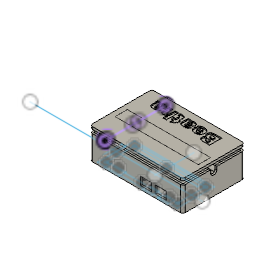
beatha (Autodesk Fusion 360 design; units mm, degrees)
Autodesk Fusion 360 part; units mm, degrees
note: some values were not read from the file. Chosen so that the rebuilt part matches the saved one: which face or edge a step refers to; which pieces of a blend or face edit are solid. Set by a fixed rule: which sketch regions a step uses.
sketch "pi w reference" plane through (0, 0, 0) normal (0, 1, 0) x (1, 0, 0)
  line L0 (-7.686, 3.5496) -> (57.314, 3.5496)
  line L1 (57.314, 3.5496) -> (57.314, -26.4504)
  line L2 (57.314, -26.4504) -> (-7.686, -26.4504)
  line L3 (-7.686, -26.4504) -> (-7.686, 3.5496)
  line L4 (-4.186, 0.0496) -> (53.814, 0.0496)
  line L5 (53.814, 0.0496) -> (53.814, -22.9504)
  line L6 (53.814, -22.9504) -> (-4.186, -22.9504)
  line L7 (-4.186, -22.9504) -> (-4.186, 0.0496)
  line L8 (24.814, 19.4382) -> (24.814, -12.339)
  line L9 (-77.996, -11.4504) -> (62.624, -11.4504)
  circle A0 centre (-4.186, 0.0496) radius 1.25
  circle A1 centre (-4.186, -22.9504) radius 1.25
  circle A2 centre (53.814, -22.9504) radius 1.25
  circle A3 centre (53.814, 0.0496) radius 1.25
  line L10 (-7.686, -3.9504) -> (-10.686, -3.9504)
  line L11 (-10.686, -3.9504) -> (-10.686, -18.9504)
  line L12 (-10.686, -18.9504) -> (-7.686, -18.9504) construction
  line L13 (-7.686, -18.9504) -> (-7.686, -3.9504)
  line L14 (-1.286, -21.9504) -> (10.714, -21.9504)
  line L15 (10.714, -21.9504) -> (10.714, -27.4504)
  line L16 (10.714, -27.4504) -> (-1.286, -27.4504)
  line L17 (-1.286, -27.4504) -> (-1.286, -21.9504)
  line L18 (29.714, -21.9504) -> (37.714, -21.9504)
  line L19 (37.714, -21.9504) -> (37.714, -27.4504)
  line L20 (37.714, -27.4504) -> (29.714, -27.4504)
  line L21 (29.714, -27.4504) -> (29.714, -21.9504)
  line L22 (42.314, -21.9504) -> (50.314, -21.9504)
  line L23 (50.314, -21.9504) -> (50.314, -27.4504)
  line L24 (50.314, -27.4504) -> (42.314, -27.4504)
  line L25 (42.314, -27.4504) -> (42.314, -21.9504)
  line L26 (-0.686, 2.1496) -> (50.314, 2.1496)
  line L27 (50.314, 2.1496) -> (50.314, -2.9504)
  line L28 (50.314, -2.9504) -> (-0.686, -2.9504)
  line L29 (-0.686, -2.9504) -> (-0.686, 2.1496)
  point P0 (53.814, -11.4504)
  point P1 (24.814, -22.9504)
  point P2 (-7.686, -11.4504)
  point P3 (4.714, -21.9504)
  point P4 (33.714, -21.9504)
  point P5 (46.314, -21.9504)
  point P6 (24.814, -2.9504)
  dimension "d1" = 65
  dimension "d2" = 30
  dimension "d3" = 3.5
  dimension "d4" = 3.5
  dimension "d5" = 3.5
  dimension "d6" = 2.5
  dimension "d7" = 12.4
  dimension "d8" = 41.4
  dimension "d9" = 54
  dimension "d10" = 8
  dimension "d11" = 12
  dimension "d12" = 15
  dimension "d13" = 3
  dimension "d14" = 1
  dimension "d15" = 1
  dimension "d16" = 51
  dimension "d17" = 5.1
  dimension "d18" = 6.5
  constraint horizontal L0
  constraint vertical L1
  constraint horizontal L2
  constraint vertical L3
  constraint horizontal L4
  constraint vertical L5
  constraint horizontal L6
  constraint vertical L7
  constraint parallel L6 L9
  constraint midpoint L3 L9
  constraint coincident L5 P0
  constraint midpoint L5 P0
  constraint coincident L9 P0
  constraint midpoint L0 L8
  constraint coincident L6 P1
  constraint midpoint L6 P1
  constraint coincident L8 P1
  constraint vertical L8
  constraint coincident L4.start L7.end
  constraint coincident L6.end L7.start
  constraint coincident L5.end L6.start
  constraint coincident L4.end L5.start
  constraint equal A0 A3
  constraint equal A2 A3
  constraint equal A1 A2
  constraint horizontal L10
  constraint vertical L11
  constraint horizontal L12
  constraint vertical L13
  constraint horizontal L14
  constraint vertical L15
  constraint horizontal L16
  constraint vertical L17
  constraint horizontal L18
  constraint vertical L19
  constraint horizontal L20
  constraint vertical L21
  constraint horizontal L22
  constraint vertical L23
  constraint horizontal L24
  constraint vertical L25
  constraint horizontal L26
  constraint vertical L27
  constraint horizontal L28
  constraint vertical L29
  constraint collinear L14 L18
  constraint collinear L18 L22
  constraint coincident L13 P2
  constraint coincident L14 P3
  constraint midpoint L18 P4
  constraint midpoint L22 P5
  constraint midpoint L14 P3
  constraint midpoint L13 P2
  constraint midpoint L3 P2
  constraint equal L18 L22
  constraint collinear L20 L24
  constraint collinear L16 L24
  constraint coincident L28 P6
  constraint midpoint L28 P6
  constraint coincident L8 P6
  measures "d1" distance of L0.start L0.end
  measures "d2" distance of L0.start L2.end
  measures "d3" distance of L3 L7
  measures "d4" distance of L0 L4
  measures "d5" distance of L1 L5
  measures "d6" diameter of A0
  measures "d7" distance of L3 P3
  measures "d8" horizontal distance of L2.end P4
  measures "d9" distance of L3 P5
  measures "d10" distance of L23.end L24.end
  measures "d11" distance of L15.end L16.end
  measures "d12" distance of L10.end L11.end
  measures "d13" distance of L11.end L12.end
  measures "d14" distance of L6 L14
  measures "d15" distance of L2 L16
  measures "d16" distance of L26.start L26.end
  measures "d17" distance of L26.start L28.end
  measures "d18" distance of L0 L28
sketch "Sketch2" plane through (0, 0, 0) normal (0, 1, 0) x (1, 0, 0)
  line L0 (-10.686, 6.5496) -> (62.314, 6.5496)
  line L1 (62.314, 6.5496) -> (62.314, -26.9504)
  line L2 (62.314, -26.9504) -> (-10.686, -26.9504)
  line L3 (-10.686, -26.9504) -> (-10.686, 6.5496)
  line L4 (57.314, 3.5496) -> (57.314, -26.4504)
  line L5 (57.314, -26.4504) -> (-7.686, -26.4504)
  line L6 (-7.686, 3.5496) -> (57.314, 3.5496)
  line L7 (-10.186, 22.1496) -> (61.814, 22.1496)
  line L8 (63.814, 20.1496) -> (63.814, -26.4504)
  line L9 (61.814, -28.4504) -> (-10.186, -28.4504)
  line L10 (-12.186, -26.4504) -> (-12.186, 20.1496)
  line L11 (-0.686, 2.1496) -> (50.314, 2.1496)
  arc A0 (-10.186, 22.1496) -> (-12.186, 20.1496) centre (-10.186, 20.1496) ccw
  arc A1 (63.814, 20.1496) -> (61.814, 22.1496) centre (61.814, 20.1496) ccw
  arc A2 (61.814, -28.4504) -> (63.814, -26.4504) centre (61.814, -26.4504) ccw
  arc A3 (-12.186, -26.4504) -> (-10.186, -28.4504) centre (-10.186, -26.4504) ccw
  point P0 (-10.686, -3.9504)
  dimension "d19" = 5
  dimension "d20" = 0.5
  dimension "d21" = 3
  dimension "d23" = 20
  dimension "d24" = 1.5
  dimension "d25" = 1.5
  dimension "d26" = 1.5
  dimension "d27" = 2
  dimension "d28" = 2
  dimension "d29" = 2
  constraint horizontal L0
  constraint vertical L1
  constraint horizontal L2
  constraint vertical L3
  constraint coincident L3 P0
  constraint horizontal L7
  constraint vertical L8
  constraint horizontal L9
  constraint vertical L10
  constraint tangent L7 A0
  constraint tangent L10 A0
  constraint tangent L7 A1
  constraint tangent L8 A1
  constraint tangent L8 A2
  constraint tangent L9 A2
  constraint equal A1 A2
  constraint tangent L9 A3
  constraint tangent L10 A3
  measures "d19" distance of L1 L4
  measures "d20" distance of L2 L5
  measures "d21" distance of L0 L6
  measures "d23" distance of L7 L11
  measures "d24" distance of L3 L10
  measures "d25" distance of L2 L9
  measures "d26" distance of L1 L8
  measures "d27" radius of A0
  measures "d28" radius of A1
  measures "d29" radius of A3
extrude "Extrude1" add sketch "Sketch2" along normal blind 20 contours L0 L1 L2 L3 | L7 L8 L9 L10 A0 A1 A2 A3 makes body 1
shell "Shell1" thickness 1.5 removed faces 1 at (37.814, 20, 11.5837) on bodies 1
extrude "Extrude2" add sketch "Sketch2" along normal blind 2 from surface at 1.5 bodies 1
sketch "Sketch4" plane through (0, 0, 28.4504) normal (0, 0, 1) x (1, 0, 0)
  line L0 (-10.186, 0) -> (61.814, 0)
  line L1 (61.814, 0) -> (61.814, 20)
  line L2 (61.814, 20) -> (-10.186, 20)
  line L3 (-10.186, 20) -> (-10.186, 0)
  line L4 (29.218, 9.4681) -> (38.218, 9.4681)
  line L5 (38.218, 9.4681) -> (38.218, 2.8854)
  line L6 (38.218, 2.8854) -> (29.218, 2.8854)
  line L7 (29.218, 2.8854) -> (29.218, 9.4681)
  line L8 (41.218, 9.4681) -> (50.218, 9.4681)
  line L9 (50.218, 9.4681) -> (50.218, 2.8854)
  line L10 (50.218, 2.8854) -> (41.218, 2.8854)
  line L11 (41.218, 2.8854) -> (41.218, 9.4681)
  line L12 (61.814, 1.5) -> (-10.186, 1.5)
  point P0 (33.718, 9.4681)
  point P1 (45.718, 9.4681)
  dimension "d39" = 9
  dimension "d128" = 12
  constraint horizontal L4
  constraint vertical L5
  constraint horizontal L6
  constraint vertical L7
  constraint horizontal L8
  constraint vertical L9
  constraint horizontal L10
  constraint vertical L11
  constraint midpoint L4 P0
  constraint coincident L8 P1
  constraint midpoint L8 P1
  constraint equal L4 L8
  constraint collinear L4 L8
  constraint collinear L6 L10
  measures "d39" distance of L8.start L8.end
  measures "d128" distance of P0 P1
extrude "Extrude3" cut sketch "Sketch4" against normal blind 3 contours L4 L5 L6 L7 | L8 L9 L10 L11 bodies 1
sketch "Sketch5" plane through (0, 0, 0) normal (0, -1, 0) x (1, 0, 0)
  arc A0 (-12.186, -20.1496) -> (-10.186, -22.1496) centre (-10.186, -20.1496) ccw
  line L0 (-10.186, -22.1496) -> (61.814, -22.1496)
  arc A1 (61.814, -22.1496) -> (63.814, -20.1496) centre (61.814, -20.1496) ccw
  line L1 (63.814, -20.1496) -> (63.814, 26.4504)
  arc A2 (63.814, 26.4504) -> (61.814, 28.4504) centre (61.814, 26.4504) ccw
  line L2 (61.814, 28.4504) -> (-10.186, 28.4504)
  arc A3 (-10.186, 28.4504) -> (-12.186, 26.4504) centre (-10.186, 26.4504) ccw
  line L3 (-12.186, 26.4504) -> (-12.186, -20.1496)
  line L4 (-14.1134, 18.9504) -> (-8.0801, 18.9504)
  line L5 (-6.0801, 16.9504) -> (-6.0801, 5.9504)
  line L6 (-8.0801, 3.9504) -> (-14.1134, 3.9504)
  line L7 (-14.1134, 3.9504) -> (-14.1134, 18.9504)
  arc A4 (-6.0801, 16.9504) -> (-8.0801, 18.9504) centre (-8.0801, 16.9504) ccw
  arc A5 (-8.0801, 3.9504) -> (-6.0801, 5.9504) centre (-8.0801, 5.9504) ccw
  point P0 (-7.686, 18.9504)
  point P1 (-7.686, 3.9504)
  dimension "d46" = 2
  constraint horizontal L4
  constraint vertical L5
  constraint horizontal L6
  constraint vertical L7
  constraint coincident L4 P0
  constraint coincident L6 P1
  constraint tangent L4 A4
  constraint tangent L5 A4
  constraint tangent L5 A5
  constraint tangent L6 A5
  constraint equal A4 A5
  measures "d46" radius of A4
extrude "Extrude4" cut sketch "Sketch5" against normal blind 3 contours L3 L4 L6 L7 | L3 L4 L5 L6 A4 A5 bodies 1
sketch "Sketch6" plane through (-12.186, 0, 0) normal (-1, 0, 0) x (0, 0, 1)
  line L0 (18.9504, 3) -> (18.9504, 0)
  line L1 (18.9504, 0) -> (26.4504, 0)
  line L2 (26.4504, 0) -> (26.4504, 20)
  line L3 (26.4504, 20) -> (-20.1496, 20)
  line L4 (-20.1496, 20) -> (-20.1496, 0)
  line L5 (-20.1496, 0) -> (3.9504, 0)
  line L6 (3.9504, 0) -> (3.9504, 3)
  line L7 (3.9504, 3) -> (18.9504, 3)
  line L8 (3.9504, 0) -> (18.9504, 0)
  line L9 (18.9504, 0) -> (18.9504, 4)
  line L10 (16.9504, 6) -> (5.9504, 6)
  line L11 (3.9504, 4) -> (3.9504, 0)
  arc A0 (5.9504, 6) -> (3.9504, 4) centre (5.9504, 4) ccw
  arc A1 (18.9504, 4) -> (16.9504, 6) centre (16.9504, 4) ccw
  dimension "d49" = 3
  dimension "d50" = 2
  constraint horizontal L8
  constraint vertical L9
  constraint horizontal L10
  constraint vertical L11
  constraint coincident L6 L5.end
  constraint coincident L0.start L9
  constraint coincident L5 L6.start
  constraint tangent L10 A0
  constraint tangent L11 A0
  constraint tangent L9 A1
  constraint tangent L10 A1
  constraint equal A0 A1
  measures "d49" distance of L7 L10
  measures "d50" radius of A0
extrude "Extrude5" cut sketch "Sketch6" against normal blind 2.873 contours L7 L9 L10 L11 A0 A1 bodies 1
extrude "Extrude6" add sketch "pi w reference" along normal blind 4 from surface at 1.5 contours L6 L7 A1 | L6 L7 A1 | L4 L7 A0 | L4 L7 A0 | L4 L5 A3 | L4 L5 A3 | L5 L6 A2 | L5 L6 A2 bodies 1
sketch "Sketch7" plane through (0, 3.5, 0) normal (0, 1, 0) x (-1, 0, 0)
  line L0 (10.686, -20.1496) -> (10.686, -6.5496)
  line L1 (10.686, -6.5496) -> (-62.314, -6.5496)
  line L2 (-62.314, -6.5496) -> (-62.314, -20.1496)
  line L3 (-13.314, -14.1496) -> (-38.314, -14.1496) construction
  line L4 (-38.314, -14.1496) -> (-38.314, -10.8331) construction
  line L5 (-38.314, -10.8331) -> (-13.314, -10.8331) construction
  line L6 (-13.314, -10.8331) -> (-13.314, -14.1496) construction
  line L7 (-25.814, -42.5951) -> (-25.814, 15.6124) construction
  line L8 (10.686, -12.4914) -> (-62.314, -12.4914) construction
  line L9 (-62.314, -20.1496) -> (-62.314, 26.4504)
  line L10 (10.686, 26.4504) -> (10.686, -20.1496)
  line L11 (-21.714, -13.4914) -> (-29.914, -13.4914)
  line L12 (-29.914, -13.4914) -> (-29.914, -11.4914)
  line L13 (-29.914, -11.4914) -> (-21.714, -11.4914)
  line L14 (-21.714, -11.4914) -> (-21.714, -13.4914)
  line L15 (10.186, -20.6496) -> (-61.814, -20.6496)
  line L16 (-21.714, -16.4914) -> (-29.914, -16.4914)
  line L17 (-29.914, -16.4914) -> (-29.914, -8.4914)
  line L18 (-29.914, -8.4914) -> (-21.714, -8.4914)
  line L19 (-21.714, -8.4914) -> (-21.714, -16.4914)
  line L20 (-21.714, -8.4914) -> (-13.4031, -8.4914)
  line L21 (-13.4031, -8.4914) -> (-13.4031, -10.9914)
  line L22 (-13.4031, -10.9914) -> (-21.714, -10.9914)
  line L23 (-21.714, -10.9914) -> (-21.714, -8.4914)
  line L24 (-38.2249, -8.4914) -> (-38.2249, -10.9914)
  line L25 (-38.2249, -10.9914) -> (-29.914, -10.9914)
  line L26 (-29.914, -8.4914) -> (-38.2249, -8.4914)
  arc A0 (-62.314, -20.1496) -> (-61.814, -20.6496) centre (-61.814, -20.1496) ccw
  line L27 (-61.814, -20.6496) -> (10.186, -20.6496)
  arc A1 (10.186, -20.6496) -> (10.686, -20.1496) centre (10.186, -20.1496) ccw
  point P0 (-25.814, -14.1496)
  point P1 (-25.814, -12.4914)
  point P2 (-38.314, -12.4914)
  point P3 (-29.914, -12.4914)
  point P4 (-21.714, -12.4914)
  point P5 (-29.914, -12.4914)
  point P6 (-38.314, -10.8331)
  dimension "d56" = 25
  dimension "d57" = 8.2
  dimension "d58" = 2
  dimension "d59" = 6.5
  dimension "d60" = 3
  dimension "d62" = 1.5
  constraint horizontal L3
  constraint vertical L4
  constraint horizontal L5
  constraint vertical L6
  constraint vertical L7
  constraint coincident L3 P0
  constraint midpoint L3 P0
  constraint coincident L7 P0
  constraint coincident L8.end L9
  constraint coincident L8.start L10
  constraint coincident L8 P1
  constraint midpoint L8 P1
  constraint coincident L7 P1
  constraint midpoint L4 P2
  constraint coincident L8 P2
  constraint horizontal L11
  constraint vertical L12
  constraint horizontal L13
  constraint vertical L14
  constraint midpoint L7 L11
  constraint coincident L12 P5
  constraint midpoint L12 P5
  constraint coincident L8 P5
  constraint horizontal L16
  constraint vertical L17
  constraint horizontal L18
  constraint vertical L19
  constraint coincident L19 P4
  constraint coincident L17 P5
  constraint midpoint L19 P4
  constraint midpoint L17 P5
  constraint collinear L12 L17
  constraint collinear L14 L19
  constraint horizontal L20
  constraint vertical L21
  constraint horizontal L22
  constraint vertical L23
  constraint symmetric L5.end L7 P6
  constraint symmetric L7 L18.end L17.end
  constraint symmetric L7 L20.end L24.start
  constraint symmetric L7 L21.end L24.end
  constraint symmetric L7 L22.end L25.end
  measures "d56" distance of L3.start L3.end
  measures "d57" distance of L11.start L11.end
  measures "d58" distance of L11.end L12.end
  measures "d59" distance of L3.start L15
  measures "d60" distance of L13 L18
  measures "d62" distance of L8 L22
extrude "Extrude7" add sketch "Sketch7" along normal blind 9 contours L11 L16 L17 L19 | L13 L17 L18 L19 L23 | L19 L20 L21 L22 L23 | L17 L24 L25 L26 bodies 1
sketch "Sketch8" plane through (0, 0, -22.1496) normal (0, 0, -1) x (-1, 0, 0)
  line L0 (-61.814, 0) -> (10.186, 0)
  line L1 (10.186, 0) -> (10.186, 20)
  line L2 (10.186, 20) -> (-61.814, 20)
  line L3 (-61.814, 20) -> (-61.814, 0)
  line L4 (-25.814, 20) -> (-25.814, -11.3409) construction
  line L5 (-40.914, 11) -> (-30.914, 11)
  line L6 (-30.914, 11) -> (-30.914, 5)
  line L7 (-30.914, 5) -> (-40.914, 5)
  line L8 (-40.914, 5) -> (-40.914, 11)
  line L9 (-29.914, 3.5) -> (-29.914, 12.5)
  line L10 (-40.914, 10.3) -> (-32.614, 10.3)
  line L11 (-31.614, 9.3) -> (-31.614, 6.7)
  line L12 (-32.614, 5.7) -> (-40.914, 5.7)
  line L13 (-40.914, 5.7) -> (-40.914, 10.3)
  arc A0 (-32.614, 5.7) -> (-31.614, 6.7) centre (-32.614, 6.7) ccw
  arc A1 (-31.614, 9.3) -> (-32.614, 10.3) centre (-32.614, 9.3) ccw
  line L14 (-40.414, 10.3) -> (-38.914, 10.3)
  line L15 (-38.914, 10.3) -> (-38.914, 5.7)
  line L16 (-38.914, 5.7) -> (-40.414, 5.7)
  line L17 (-40.414, 5.7) -> (-40.414, 10.3)
  line L18 (-12.714, 10.3) -> (-12.714, 5.7)
  line L19 (-10.714, 10.3) -> (-19.014, 10.3)
  line L20 (-20.014, 9.3) -> (-20.014, 6.7)
  line L21 (-11.214, 10.3) -> (-12.714, 10.3)
  line L22 (-20.714, 5) -> (-10.714, 5)
  line L23 (-19.014, 5.7) -> (-10.714, 5.7)
  line L24 (-11.214, 5.7) -> (-11.214, 10.3)
  line L25 (-10.714, 5.7) -> (-10.714, 10.3)
  line L26 (-10.714, 11) -> (-20.714, 11)
  line L27 (-20.714, 11) -> (-20.714, 5)
  arc A2 (-20.014, 6.7) -> (-19.014, 5.7) centre (-19.014, 6.7) ccw
  arc A3 (-19.014, 10.3) -> (-20.014, 9.3) centre (-19.014, 9.3) ccw
  line L28 (-12.714, 5.7) -> (-11.214, 5.7)
  line L29 (-10.714, 5) -> (-10.714, 11)
  circle A4 centre (-31.6227, 8) radius 0.0087
  circle A5 centre (-20.0053, 8) radius 0.0087
  line L30 (-10.714, 8) -> (-40.914, 8) construction
  point P0 (-40.914, 8)
  point P1 (-21.714, 12.5)
  point P2 (-10.714, 8)
  point P3 (-21.714, 3.5)
  dimension "d66" = 1
  dimension "d68" = 6
  dimension "d69" = 10
  dimension "d70" = 0.7
  dimension "d71" = 0.7
  dimension "d72" = 1
  dimension "d73" = 0.5
  dimension "d74" = 1.5
  constraint coincident L2 L4.start
  constraint midpoint L2 L4.start
  constraint vertical L4
  constraint horizontal L5
  constraint vertical L6
  constraint horizontal L7
  constraint vertical L8
  constraint horizontal L10
  constraint vertical L11
  constraint horizontal L12
  constraint vertical L13
  constraint coincident L13 P0
  constraint midpoint L13 P0
  constraint midpoint L8 P0
  constraint tangent L11 A0
  constraint tangent L12 A0
  constraint tangent L10 A1
  constraint tangent L11 A1
  constraint equal A0 A1
  constraint horizontal L14
  constraint vertical L15
  constraint horizontal L16
  constraint vertical L17
  constraint coincident L12 L15.end
  constraint coincident L10 L14.start
  constraint symmetric L4 L5.start L26.start
  constraint symmetric L4 L5.end L26.end
  constraint symmetric L4 L6.end L22.start
  constraint symmetric L4 L7.end L22.end
  constraint symmetric L4 L9.start P3
  constraint symmetric L4 L9.end P1
  constraint symmetric L4 L10.start L19.start
  constraint symmetric L4 L12.end L23.end
  constraint symmetric L4 P0 P2
  constraint symmetric L4 L11.end L20.end
  constraint symmetric L4 L12.start L23.start
  constraint symmetric L4 A0 A2
  constraint symmetric L4 L10.end L19.end
  constraint symmetric L4 L11.start L20.start
  constraint symmetric L4 A1 A3
  constraint symmetric L4 L14.start L21.start
  constraint symmetric L4 L14.end L18.start
  constraint symmetric L4 L15.end L18.end
  constraint symmetric L4 L16.end L24.start
  constraint coincident P2 L30.start
  constraint coincident P0 L30.end
  constraint coincident A4.centre L30
  constraint coincident A5.centre L30
  constraint equal A4 A5
  constraint tangent L11 A4
  constraint tangent L20 A5
  measures "d66" distance of L5.end L9
  measures "d68" distance of L5 L7
  measures "d69" distance of L5.start L5.end
  measures "d70" distance of L5 L10
  measures "d71" distance of L6 L11
  measures "d72" radius of A0
  measures "d73" distance of L8 L17
  measures "d74" distance of L15 L17
extrude "Extrude8" cut sketch "Sketch8" against normal blind 1.5 draft -1 contours L5 L6 L7 L8 L10 L11 L12 A0 A1 L14 L16 | L19 L20 L21 L22 L23 L26 L27 A2 A3 L28 L29 bodies 1
extrude "Extrude9" cut sketch "Sketch8" against normal blind 0.75 draft -25 contours L10 L12 L14 L15 L16 L17 | L18 L19 L21 L23 L24 L28 bodies 1
extrude "Extrude10" add sketch "Sketch8" along normal blind 1.5 draft -15 contours A4 | A5 bodies 1
sketch "Sketch9" plane through (63.814, 0, 0) normal (1, 0, 0) x (0, 0, -1)
  line L0 (-26.4504, 0) -> (20.1496, 0)
  line L1 (20.1496, 0) -> (20.1496, 20)
  line L2 (20.1496, 20) -> (-26.4504, 20)
  line L3 (-26.4504, 20) -> (-26.4504, 0)
  line L4 (-5.6504, 20) -> (-0.6504, 20)
  line L5 (-0.6504, 20) -> (-0.6504, 15)
  line L6 (-0.6504, 15) -> (-5.6504, 15)
  line L7 (-5.6504, 15) -> (-5.6504, 20)
  line L8 (-3.1504, 20) -> (-3.1504, 10) construction
  circle A0 centre (-3.1504, 17.5) radius 2.5
  dimension "d81" = 5
  dimension "d82" = 5
  constraint horizontal L4
  constraint vertical L5
  constraint horizontal L6
  constraint vertical L7
  constraint perpendicular L6 L8
  constraint midpoint L2 L8.start
  constraint midpoint L6 L8
  constraint collinear L2 L4
  constraint tangent L6 A0
  constraint tangent L5 A0
  constraint tangent L7 A0
  measures "d81" distance of L2 L6
  measures "d82" distance of L5.end L6.end
extrude "Extrude11" cut sketch "Sketch9" against normal blind 4.015 contours L2 L4 L7 A0 | L2 L4 L5 A0 | A0 bodies 1
sketch "Sketch11" plane through (0, 0, 0) normal (1, 0, 0) x (0, 0, -1)
  line L0 (-26.4504, 20) -> (20.1496, 20)
  line L1 (-5.6504, 20) -> (-26.4504, 20)
  line L2 (-26.9504, 20) -> (-26.4504, 20)
  line L3 (-26.9504, 20) -> (-26.4504, 20)
  line L4 (-26.4504, 20) -> (20.1496, 20)
  line L5 (20.1496, 20) -> (20.6496, 20)
  line L6 (20.1496, 20) -> (20.6496, 20)
  line L7 (20.1496, 20) -> (-0.6504, 20)
  line L8 (-0.6504, 20) -> (20.1496, 20)
  line L9 (22.1496, 20) -> (20.1496, 20)
  line L10 (22.1496, 20) -> (20.1496, 20)
  line L11 (20.1496, 20) -> (-26.4504, 20)
  line L12 (-26.4504, 20) -> (-28.4504, 20)
  line L13 (-26.4504, 20) -> (-28.4504, 20)
  line L14 (-26.4504, 20) -> (-5.6504, 20)
extrude "Extrude13" add 1 faces at (37.814, 20, -21.1496) along direction (0, 1, 0) blind 2 from surface at 3 on bodies 1 bodies 1 makes body 2
sketch "Sketch12" plane through (0, 23, 0) normal (0, -1, 0) x (1, 0, 0)
  line L0 (62.314, 5.6504) -> (63.814, 5.6504) construction
  line L1 (63.814, 5.6504) -> (63.814, 26.4504)
  arc A0 (63.814, 26.4504) -> (61.814, 28.4504) centre (61.814, 26.4504) ccw
  line L2 (61.814, 28.4504) -> (-10.186, 28.4504)
  arc A1 (-10.186, 28.4504) -> (-12.186, 26.4504) centre (-10.186, 26.4504) ccw
  line L3 (-12.186, 26.4504) -> (-12.186, -20.1496)
  arc A2 (-12.186, -20.1496) -> (-10.186, -22.1496) centre (-10.186, -20.1496) ccw
  line L4 (-10.186, -22.1496) -> (61.814, -22.1496)
  arc A3 (61.814, -22.1496) -> (63.814, -20.1496) centre (61.814, -20.1496) ccw
  line L5 (63.814, -20.1496) -> (63.814, 0.6504)
  line L6 (63.814, 0.6504) -> (62.314, 0.6504) construction
  line L7 (62.314, 0.6504) -> (62.314, -20.1496) construction
  arc A4 (61.814, -20.6496) -> (62.314, -20.1496) centre (61.814, -20.1496) ccw construction
  line L8 (61.814, -20.6496) -> (-10.186, -20.6496) construction
  arc A5 (-10.686, -20.1496) -> (-10.186, -20.6496) centre (-10.186, -20.1496) ccw construction
  line L9 (-10.686, -20.1496) -> (-10.686, 26.4504) construction
  arc A6 (-10.186, 26.9504) -> (-10.686, 26.4504) centre (-10.186, 26.4504) ccw construction
  line L10 (-10.186, 26.9504) -> (61.814, 26.9504) construction
  arc A7 (62.314, 26.4504) -> (61.814, 26.9504) centre (61.814, 26.4504) ccw construction
  line L11 (62.314, 26.4504) -> (62.314, 5.6504) construction
  line L12 (60.064, -20.4496) -> (-8.286, -20.4496)
  line L13 (-10.286, -18.4496) -> (-10.286, 24.3504)
  line L14 (-8.286, 26.3504) -> (60.064, 26.3504)
  line L15 (62.064, 24.3504) -> (62.064, -18.4496)
  line L16 (25.814, -22.1496) -> (25.814, 28.4504) construction
  line L17 (-12.186, 3.1504) -> (62.064, 3.1504) construction
  line L18 (61.814, -22.1496) -> (-10.186, -22.1496)
  line L19 (-12.186, -20.1496) -> (-12.186, 26.4504)
  line L20 (-10.186, 28.4504) -> (61.814, 28.4504)
  line L21 (63.814, 26.4504) -> (63.814, -20.1496)
  line L22 (62.314, 0.6504) -> (63.814, 0.6504)
  line L23 (63.814, 0.6504) -> (63.814, 5.6504)
  line L24 (63.814, 5.6504) -> (62.314, 5.6504)
  line L25 (62.314, 5.6504) -> (62.314, 0.6504)
  arc A8 (61.814, -22.1496) -> (63.814, -20.1496) centre (61.814, -20.1496) ccw
  arc A9 (63.814, 26.4504) -> (61.814, 28.4504) centre (61.814, 26.4504) ccw
  arc A10 (62.064, 24.3504) -> (60.064, 26.3504) centre (60.064, 24.3504) ccw
  arc A11 (60.064, -20.4496) -> (62.064, -18.4496) centre (60.064, -18.4496) ccw
  arc A12 (-10.186, 28.4504) -> (-12.186, 26.4504) centre (-10.186, 26.4504) ccw
  arc A13 (-8.286, 26.3504) -> (-10.286, 24.3504) centre (-8.286, 24.3504) ccw
  arc A14 (-10.286, -18.4496) -> (-8.286, -20.4496) centre (-8.286, -18.4496) ccw
  arc A15 (-12.186, -20.1496) -> (-10.186, -22.1496) centre (-10.186, -20.1496) ccw
  point P0 (25.814, -20.4496)
  point P1 (62.064, 2.9504)
  dimension "d91" = 0.2
  dimension "d92" = 0.25
  dimension "d93" = 2
  constraint horizontal L12
  constraint vertical L13
  constraint horizontal L14
  constraint vertical L15
  constraint midpoint L4 L16.start
  constraint midpoint L2 L16.end
  constraint coincident L12 P0
  constraint coincident L15 P1
  constraint coincident L16 P0
  constraint coincident L3 L17.start
  constraint horizontal L17
  constraint midpoint L3 L17.start
  constraint horizontal L18
  constraint vertical L19
  constraint horizontal L20
  constraint vertical L21
  constraint collinear L4 L18
  constraint collinear L5 L21
  constraint collinear L2 L20
  constraint collinear L3 L19
  constraint horizontal L22
  constraint vertical L23
  constraint horizontal L24
  constraint vertical L25
  constraint coincident L0.end L1.start
  constraint coincident L6.end L7.start
  constraint tangent L18 A8
  constraint tangent L21 A8
  constraint tangent L20 A9
  constraint tangent L21 A9
  constraint equal A8 A9
  constraint coincident L15 L17.end
  constraint tangent L14 A10
  constraint tangent L15 A10
  constraint equal A8 A10
  constraint tangent L12 A11
  constraint tangent L15 A11
  constraint equal A8 A11
  constraint tangent L19 A12
  constraint tangent L20 A12
  constraint equal A8 A12
  constraint tangent L13 A13
  constraint tangent L14 A13
  constraint equal A8 A13
  constraint tangent L12 A14
  constraint tangent L13 A14
  constraint equal A8 A14
  constraint tangent L18 A15
  constraint tangent L19 A15
  constraint equal A8 A15
  measures "d91" distance of L8 L12
  measures "d92" distance of L7 L15
  measures "d93" radius of A8
extrude "Extrude14" add sketch "Sketch12" against normal blind 2 contours L1 A0 L2 A1 L3 A2 L4 A3 L5 L18 L19 L20 L21 L22 L24 L25 A8 A9 A12 A15 | L21 L22 L23 L24 L25 | L12 L13 L14 L15 A10 A11 A13 A14 bodies 2
extrude "Extrude15" add sketch "Sketch12" along normal blind 1 contours L12 L13 L14 L15 A10 A11 A13 A14 bodies 2
sketch "Sketch13" plane through (0, 22, 0) normal (0, -1, 0) x (1, 0, 0)
  arc A0 (-8.286, 26.3504) -> (-10.286, 24.3504) centre (-8.286, 24.3504) ccw
  line L0 (-10.286, 24.3504) -> (-10.286, -18.4496)
  arc A1 (-10.286, -18.4496) -> (-8.286, -20.4496) centre (-8.286, -18.4496) ccw
  line L1 (-8.286, -20.4496) -> (60.064, -20.4496)
  arc A2 (60.064, -20.4496) -> (62.064, -18.4496) centre (60.064, -18.4496) ccw
  line L2 (62.064, -18.4496) -> (62.064, 24.3504)
  arc A3 (62.064, 24.3504) -> (60.064, 26.3504) centre (60.064, 24.3504) ccw
  line L3 (60.064, 26.3504) -> (-8.286, 26.3504)
  line L4 (58.2633, 0.6504) -> (52.2633, 0.6504)
  line L5 (52.2633, 0.6504) -> (52.2633, 5.6504)
  line L6 (52.2633, 5.6504) -> (58.2633, 5.6504)
  line L7 (58.2633, 5.6504) -> (58.2633, 0.6504)
  line L8 (63.814, 5.6504) -> (62.314, 5.6504)
  line L9 (62.314, 0.6504) -> (63.814, 0.6504)
  dimension "d98" = 6
  constraint horizontal L4
  constraint vertical L5
  constraint horizontal L6
  constraint vertical L7
  constraint collinear L6 L8
  constraint collinear L4 L9
  measures "d98" distance of L4.start L4.end
sketch "Sketch14" plane through (0, 1.5, 0) normal (0, 1, 0) x (-1, 0, 0)
  circle A0 centre (-53.814, 22.9504) radius 1.25
  circle A1 centre (4.186, -0.0496) radius 1.25
  circle A2 centre (-53.814, -0.0496) radius 1.25
  circle A3 centre (4.186, 22.9504) radius 1.25
  line L0 (8.0801, 18.9504) -> (10.686, 18.9504)
  line L1 (10.686, 18.9504) -> (10.686, 26.4504)
  arc A4 (10.686, 26.4504) -> (10.186, 26.9504) centre (10.186, 26.4504) ccw
  line L2 (10.186, 26.9504) -> (-61.814, 26.9504)
  arc A5 (-61.814, 26.9504) -> (-62.314, 26.4504) centre (-61.814, 26.4504) ccw
  line L3 (-62.314, 26.4504) -> (-62.314, -6.5496)
  line L4 (-62.314, -6.5496) -> (10.686, -6.5496)
  line L5 (10.686, -6.5496) -> (10.686, 3.9504)
  line L6 (10.686, 3.9504) -> (8.0801, 3.9504)
  arc A6 (6.0801, 5.9504) -> (8.0801, 3.9504) centre (8.0801, 5.9504) ccw
  line L7 (6.0801, 5.9504) -> (6.0801, 16.9504)
  arc A7 (8.0801, 18.9504) -> (6.0801, 16.9504) centre (8.0801, 16.9504) ccw
  circle A8 centre (4.186, 22.9504) radius 2.45
  circle A9 centre (4.186, -0.0496) radius 2.45
  circle A10 centre (-53.814, -0.0496) radius 2.45
  circle A11 centre (-53.814, 22.9504) radius 2.45
  circle A12 centre (4.186, 22.9504) radius 1.25
  dimension "d99" = 1.2
  constraint concentric A3 A8
  constraint concentric A1 A9
  constraint concentric A2 A10
  constraint concentric A0 A11
  constraint equal A8 A11
  constraint equal A8 A9
  constraint equal A9 A10
  measures "d99" distance of A8 A12
extrude "Extrude16" add sketch "Sketch14" along normal blind 2.5 contours A8 | A9 | A10 | A11 bodies 1
sketch "Sketch19" plane through (0, 3.5, 0) normal (0, 1, 0) x (-1, 0, 0)
  line L0 (-13.4031, -8.4914) -> (-13.4031, -10.9914)
  line L1 (-13.4031, -10.9914) -> (-21.714, -10.9914)
  line L2 (-21.714, -10.9914) -> (-21.714, -11.4914)
  line L3 (-21.714, -11.4914) -> (-29.914, -11.4914)
  line L4 (-29.914, -11.4914) -> (-29.914, -10.9914)
  line L5 (-29.914, -10.9914) -> (-38.2249, -10.9914)
  line L6 (-38.2249, -10.9914) -> (-38.2249, -8.4914)
  line L7 (-38.2249, -8.4914) -> (-13.4031, -8.4914)
  line L8 (-21.714, -16.4914) -> (-29.914, -16.4914)
  line L9 (-29.914, -16.4914) -> (-29.914, -13.4914)
  line L10 (-29.914, -13.4914) -> (-21.714, -13.4914)
  line L11 (-21.714, -13.4914) -> (-21.714, -16.4914)
  line L12 (-62.314, -6.5496) -> (-62.314, -20.1496)
  arc A0 (-62.314, -20.1496) -> (-61.814, -20.6496) centre (-61.814, -20.1496) ccw
  line L13 (-61.814, -20.6496) -> (10.186, -20.6496)
  arc A1 (10.186, -20.6496) -> (10.686, -20.1496) centre (10.186, -20.1496) ccw
  line L14 (10.686, -20.1496) -> (10.686, -6.5496)
  line L15 (10.686, -6.5496) -> (-62.314, -6.5496)
  line L16 (-56.2223, -4.9732) -> (-41.2673, -4.9732)
  line L17 (-41.2673, -4.9732) -> (-41.2673, -12.8035)
  line L18 (-41.2673, -12.8035) -> (-56.2223, -12.8035)
  line L19 (-56.2223, -12.8035) -> (-56.2223, -4.9732)
  constraint horizontal L16
  constraint vertical L17
  constraint horizontal L18
  constraint vertical L19
extrude "Extrude20" cut sketch "Sketch19" against normal blind 2 contours L15 L17 L18 L19 bodies 1
fillet "Fillet4" radius 3 3 edges at (56.2223, 3.5, -9.6765) (48.7448, 3.5, -12.8035) (41.2673, 3.5, -9.6765) on bodies 1
fillet "Fillet1" radius 1.5 5 edges at (-9.3831, 1.5, 3.9504) (-6.6659, 1.5, 4.5362) (-6.0801, 1.5, 11.4504) (-6.6659, 1.5, 18.3646) (-9.3831, 1.5, 18.9504) on bodies 1
fillet "Fillet3" radius 0.8 2 faces at (39.5306, 7.3499, -21.3996) (11.8306, 8.6501, -21.3996) on bodies 1
sketch "Sketch16" plane through (0, 25, 0) normal (0, 1, 0) x (-1, 0, 0)
  line L0 (-63.814, 26.4504) -> (-63.814, -20.1496)
  arc A0 (-63.814, -20.1496) -> (-61.814, -22.1496) centre (-61.814, -20.1496) ccw
  line L1 (-61.814, -22.1496) -> (10.186, -22.1496)
  arc A1 (10.186, -22.1496) -> (12.186, -20.1496) centre (10.186, -20.1496) ccw
  line L2 (12.186, -20.1496) -> (12.186, 26.4504)
  arc A2 (12.186, 26.4504) -> (10.186, 28.4504) centre (10.186, 26.4504) ccw
  line L3 (10.186, 28.4504) -> (-61.814, 28.4504)
  arc A3 (-61.814, 28.4504) -> (-63.814, 26.4504) centre (-61.814, 26.4504) ccw
  line L4 (-59.814, 11.817) -> (8.186, 11.817)
  line L5 (8.186, 11.817) -> (8.186, 1.817)
  line L6 (8.186, 1.817) -> (-59.814, 1.817)
  line L7 (-59.814, 1.817) -> (-59.814, 11.817)
  line L8 (-25.814, -22.1496) -> (-25.814, 1.817) construction
  dimension "d111" = 68
  dimension "d112" = 10
  constraint horizontal L4
  constraint vertical L5
  constraint horizontal L6
  constraint vertical L7
  constraint coincident L1 L8.start
  constraint coincident L6 L8.end
  constraint midpoint L1 L8.start
  constraint vertical L8
  constraint midpoint L6 L8.end
  measures "d111" distance of L4.start L4.end
  measures "d112" distance of L4 L6
extrude "Extrude17" cut sketch "Sketch16" against normal blind 4 from surface at -0.4 contours L4 L5 L6 L7 bodies 2
sketch "Sketch17" plane through (0, 25, 0) normal (0, 1, 0) x (-1, 0, 0)
  line L0 (-63.814, 26.4504) -> (-63.814, -20.1496)
  arc A0 (-63.814, -20.1496) -> (-61.814, -22.1496) centre (-61.814, -20.1496) ccw
  line L1 (-61.814, -22.1496) -> (10.186, -22.1496)
  arc A1 (10.186, -22.1496) -> (12.186, -20.1496) centre (10.186, -20.1496) ccw
  line L2 (12.186, -20.1496) -> (12.186, 26.4504)
  arc A2 (12.186, 26.4504) -> (10.186, 28.4504) centre (10.186, 26.4504) ccw
  line L3 (10.186, 28.4504) -> (-61.814, 28.4504)
  arc A3 (-61.814, 28.4504) -> (-63.814, 26.4504) centre (-61.814, 26.4504) ccw
  line L4 (-50.8338, -6.8128) -> (1.1561, -7.1921) construction
  line L5 (1.1561, -7.1921) -> (1.1603, -6.6168) construction
  line L6 (1.1603, -6.6168) -> (-50.8296, -6.2375) construction
  line L7 (-50.8296, -6.2375) -> (-50.8338, -6.8128) construction
  dimension "d116" = 10
  text T0 "Beatha" font "Arial Black" height 10 align left top in box 51.9912 x 0.5753 at (-50.8338, -6.8128) x (0.999973, -0.007297) y (0.007297, 0.999973) spacing 1
extrude "Extrude18" cut sketch "Sketch17" against normal blind 1 text T0 bodies 2
sketch "Sketch18" plane through (0, 0, -22.1496) normal (0, 0, -1) x (-1, 0, 0)
  line L0 (-61.814, 20) -> (-61.814, 0)
  line L1 (-61.814, 0) -> (10.186, 0)
  line L2 (10.186, 0) -> (10.186, 20)
  line L3 (10.186, 20) -> (-61.814, 20)
  line L4 (-40.414, 5.7) -> (-40.414, 10.3)
  line L5 (-40.414, 10.3) -> (-40.914, 10.3)
  line L6 (-40.914, 10.3) -> (-40.914, 11)
  line L7 (-40.914, 11) -> (-30.914, 11)
  line L8 (-30.914, 11) -> (-30.914, 5)
  line L9 (-30.914, 5) -> (-40.914, 5)
  line L10 (-40.914, 5) -> (-40.914, 5.7)
  line L11 (-40.914, 5.7) -> (-40.414, 5.7)
  line L12 (-11.214, 10.3) -> (-11.214, 5.7)
  line L13 (-11.214, 5.7) -> (-10.714, 5.7)
  line L14 (-10.714, 5.7) -> (-10.714, 5)
  line L15 (-10.714, 5) -> (-20.714, 5)
  line L16 (-20.714, 5) -> (-20.714, 11)
  line L17 (-20.714, 11) -> (-10.714, 11)
  line L18 (-10.714, 11) -> (-10.714, 10.3)
  line L19 (-10.714, 10.3) -> (-11.214, 10.3)
  line L20 (-43.5092, 13.2964) -> (-28.4789, 13.2964) construction
  line L21 (-28.4789, 13.2964) -> (-28.4789, 16.1043) construction
  line L22 (-28.4789, 16.1043) -> (-43.5092, 16.1043) construction
  line L23 (-43.5092, 16.1043) -> (-43.5092, 13.2964) construction
  line L24 (-18.2385, 12.7183) -> (-7.3374, 12.7183) construction
  line L25 (-7.3374, 12.7183) -> (-7.3374, 16.1869) construction
  line L26 (-7.3374, 16.1869) -> (-18.2385, 16.1869) construction
  line L27 (-18.2385, 16.1869) -> (-18.2385, 12.7183) construction
  dimension "d120" = 4
  dimension "d122" = 4
  text T0 "Pair" font "Arial Black" height 4 align left top in box 15.0303 x 2.8079 at (-43.5092, 13.2964) x (1, 0) y (0, 1) spacing 1
  text T1 "BT" font "Arial Black" height 4 align left top in box 10.9011 x 3.4685 at (-18.2385, 12.7183) x (1, 0) y (0, 1) spacing 1
extrude "Extrude19" add sketch "Sketch18" along normal blind 1 text T1 T0 bodies 1
sketch "Sketch20" plane through (0, 0, -22.1496) normal (0, 0, -1) x (-1, 0, 0)
  line L0 (-38.914, 10.3) -> (-38.914, 5.7)
  line L1 (-38.914, 5.7) -> (-32.614, 5.7)
  arc A0 (-32.614, 5.7) -> (-31.614, 6.7) centre (-32.614, 6.7) ccw
  line L2 (-31.614, 6.7) -> (-31.614, 8)
  circle A1 centre (-31.6227, 8) radius 0.0087
  line L3 (-31.614, 8) -> (-31.614, 9.3)
  arc A2 (-31.614, 9.3) -> (-32.614, 10.3) centre (-32.614, 9.3) ccw
  line L4 (-32.614, 10.3) -> (-38.914, 10.3)
  circle A3 centre (-34.5114, 8) radius 2.3
  circle A4 centre (-17.1808, 8) radius 2.3
  line L5 (-12.714, 10.3) -> (-19.014, 10.3)
  line L6 (-34.5114, 8) -> (-17.1808, 8) construction
  line L7 (-19.014, 5.7) -> (-12.714, 5.7)
  constraint coincident A0.centre A3
  constraint tangent A4 L5
  constraint equal A3 A4
  constraint coincident A3.centre L6.start
  constraint coincident A4.centre L6.end
  constraint horizontal L6
  constraint tangent A4 L7
extrude "Extrude21" add sketch "Sketch20" along normal blind 1.5 contours A3 | A4 bodies 1
fillet "Fillet5" radius 1 2 faces at (33.3954, 8.605, -23.6496) (16.1782, 7.378, -23.6496) on bodies 1
equation "d117 = 'Beatha'"
equation "d121 = 'Pair'"
equation "d123 = 'BT'"
